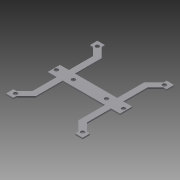
# Autodesk Inventor part: MotorSideHolder
Saved by Autodesk Inventor 2014 SP1 (Build 180222100, 222)
## iProperties
Created: 2015-03-30
Part Number: MotorSideHolder
Material: Generic
Document SubType Name: Modeling
Designer: Erin
Density: 1 g/cm^3
Appearance: Default
Author: Erin
Autodesk Inventor part; units mm, degrees
note: some values were not read from the file. Chosen so that the rebuilt part matches the saved one: sketch regions of "Extrusion1".
ref_plane "YZ Plane" through (0, 0, 0) normal (1, 0, 0) x (0, 1, 0)
ref_plane "XZ Plane" through (0, 0, 0) normal (0, 1, 0) x (-1, 0, 0)
ref_plane "XY Plane" through (0, 0, 0) normal (0, 0, 1) x (1, 0, 0)
sketch "Sketch1" plane through (0, 0, 0) normal (0, 0, 1) x (1, 0, 0)
  line L0 (-41.5, 50) -> (41.5, 50) construction
  line L1 (41.5, 50) -> (41.5, -50) construction
  line L2 (41.5, -50) -> (-41.5, -50) construction
  line L3 (-41.5, -50) -> (-41.5, 50) construction
  line L4 (0, 52.1292) -> (0, -48.3366) construction
  line L5 (-75.7124, 0) -> (96.9256, 0) construction
  circle A0 centre (-38.5, 47) radius 2.25
  line L6 (-31.25, 7) -> (0, 7)
  line L7 (0, 7) -> (0, -7)
  line L8 (0, -7) -> (-31.25, -7)
  line L9 (-31.25, -7) -> (-31.25, 7)
  circle A1 centre (-19, 0) radius 2.25
  line L10 (38.5, 47) -> (-38.5, 47) construction
  line L11 (-38.5, 47) -> (-38.5, -47) construction
  line L12 (-38.5, -47) -> (38.5, -47) construction
  line L13 (38.5, -47) -> (38.5, 47) construction
  circle A2 centre (38.5, 47) radius 2.25
  circle A3 centre (38.5, -47) radius 2.25
  circle A4 centre (-38.5, -47) radius 2.25
  line L14 (-31.25, -7) -> (-24.25, -7)
  line L15 (-24.25, -7) -> (-24.25, -37.6997)
  line L16 (-24.25, -37.6997) -> (-31.25, -37.6997)
  line L17 (-31.25, -37.6997) -> (-31.25, -7)
  line L18 (-44, -47.5503) -> (-39.0503, -52.5)
  line L19 (-39.0503, -52.5) -> (-24.25, -37.6997)
  line L20 (-24.25, -37.6997) -> (-29.1997, -32.75)
  line L21 (-29.1997, -32.75) -> (-44, -47.5503)
  line L22 (-26.7249, -35.2249) -> (-41.5251, -50.0251) construction
  line L23 (-41.5, -50) -> (-10.8193, -19.3193) construction
  line L24 (-41.5, -50) -> (1.8891, -50) construction
  line L25 (-35.5, -44) -> (-44, -44)
  line L26 (-44, -44) -> (-44, -52.5)
  line L27 (-44, -52.5) -> (-35.5, -52.5)
  line L28 (-35.5, -52.5) -> (-35.5, -44)
  circle A5 centre (-38.5, 0) radius 2.25
  line L29 (-31.25, 7) -> (-41.5, 7)
  line L30 (-41.5, 7) -> (-41.5, -7)
  line L31 (-41.5, -7) -> (-31.25, -7)
  line L32 (-31.25, -7) -> (-31.25, 7)
  point P0 (0, 0)
  point P1 (41.5, 0)
  point P2 (0, 50)
  dimension "d0" = 83
  dimension "d3" = 4.5
  dimension "d5" = 3
  dimension "d9" = 14
  dimension "d10" = 4.5
  dimension "d11" = 19
  dimension "d14" = 100
  dimension "d16" = 3
  dimension "d17" = 4.5
  dimension "d18" = 4.5
  dimension "d19" = 4.5
  dimension "d20" = 7
  dimension "d21" = 7
  dimension "d22" = 45
  dimension "d23" = 3
  dimension "d24" = 5.5
  dimension "d25" = 5.5
  dimension "d26" = 3
  dimension "d27" = 3
  dimension "d28" = 4.5
  constraints: 67 end point, 14 parallel, 8 perpendicular, 7 horizontal, 6 centre point, 5 midpoint, 5 point on line, 3 coincident, 2 collinear, 1 equal length, 1 horizontal alignment, 1 vertical, 1 vertical alignment, 3 other
  measures "d0" distance of L1.end L2.end
  measures "d3" diameter of A0
  measures "d5" distance from line of A0.centre L0
  measures "d9" distance of L6.end L7.end
  measures "d10" diameter of A1
  measures "d11" distance from line of A1.centre L4
  measures "d14" distance of L0.end L1.end
  measures "d16" distance between parallel lines of L10 L0
  measures "d17" diameter of A2
  measures "d18" diameter of A3
  measures "d19" diameter of A4
  measures "d20" distance of L15.end L16.end
  measures "d21" distance of L15.end L20.end
  measures "d22" angle of L24 L23
  measures "d23" distance edge to line of A1 L15
  measures "d24" distance from line of A4.centre L27
  measures "d25" distance from line of A4.centre L26
  measures "d26" distance from line of A4.centre L25
  measures "d27" distance from line of A4.centre L28
  measures "d28" diameter of A5
extrude "Extrusion1" add sketch "Sketch1" along normal blind 1.5 contours L6 L7 L8 L9 | L9 L31 L30 L29 | L8 L15 L20 L21 L17 | L21 L20 L16 L17 | L17 L16 L19 L28 L25 L21 | L25 L28 L19 L18 L21 | L21 L26 L25 | L28 L27 L19 | L18 L27 L26
mirror "Mirror1" about plane through (0, 0, 0) normal (1, 0, 0) of "Extrusion1"
mirror "Mirror2" about plane through (0, 0, 0) normal (0, 1, 0) of "Extrusion1", "Mirror1"
body "Solid1"
